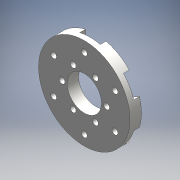
# Autodesk Inventor part: terminal-cap
Saved by Autodesk Inventor 2018 (Build 220112000, 112)
## iProperties
Created: 2026-06-13
Part Number: terminal-cap
Material: Generic
Document SubType Name: Modeling
Designer: neo
Density: 1 g/cm^3
Appearance: Default
Author: neo
Autodesk Inventor part; units mm, degrees
ref_plane "YZ Plane" through (0, 0, 0) normal (1, 0, 0) x (0, 1, 0)
ref_plane "XZ Plane" through (0, 0, 0) normal (0, 1, 0) x (-1, 0, 0)
ref_plane "XY Plane" through (0, 0, 0) normal (0, 0, 1) x (1, 0, 0)
sketch "Sketch1" plane through (0, 0, 0) normal (0, 1, 0) x (-1, 0, 0)
  circle A0 centre (0, 0) radius 30
  circle A1 centre (0, 0) radius 39 construction
  circle A2 centre (0, 0) radius 80
  circle A3 centre (39, 0) radius 5.1
  circle A4 centre (19.5, 33.775) radius 5.1
  circle A5 centre (-19.5, 33.775) radius 5.1
  circle A6 centre (-39, 0) radius 5.1
  circle A7 centre (-19.5, -33.775) radius 5.1
  circle A8 centre (19.5, -33.775) radius 5.1
  dimension "d0" = 78
  dimension "d1" = 160
  dimension "d2" = 60
  dimension "d3" = 10.2
  dimension "d6" = 360
  constraints: 8 centre point, 3 coincident, 1 horizontal alignment, 15 other
  measures "d1" diameter of A2
  measures "d2" diameter of A0
  measures "d3" diameter of A3
extrude "Extrusion1" add sketch "Sketch1" along normal blind 20
sketch "Sketch2" plane through (0, 20, 0) normal (0, 1, 0) x (1, 0, 0)
  circle A0 centre (0, 0) radius 30 construction
  circle A1 centre (-19.5, 33.775) radius 5.1 construction
  circle A2 centre (19.5, 33.775) radius 5.1 construction
  circle A3 centre (39, 0) radius 5.1 construction
  circle A4 centre (19.5, -33.775) radius 5.1 construction
  circle A5 centre (-19.5, -33.775) radius 5.1 construction
  circle A6 centre (-39, 0) radius 5.1 construction
  circle A7 centre (0, 0) radius 80 construction
  line L0 (0, -80) -> (0, 80) construction
  line L1 (-18, 80) -> (18, 80)
  line L2 (18, 80) -> (18, 44)
  line L3 (18, 44) -> (-18, 44)
  line L4 (-18, 44) -> (-18, 80)
  circle A8 centre (0, 0) radius 80 construction
  circle A9 centre (0, 62) radius 5.05
  dimension "d10" = 36
  dimension "d11" = 10.1
  dimension "d12" = 18
  dimension "d13" = 36
  constraints: 10 end point, 2 parallel, 2 point on circle, 1 centre point, 1 horizontal, 1 perpendicular, 1 point on line, 1 tangent, 1 vertical, 1 other
  measures "d10" distance between parallel lines of L2 L4
  measures "d11" diameter of A9
  measures "d12" distance from line of L1 A9.centre
  measures "d13" distance of L3.end L1.start
extrude "Extrusion2" cut sketch "Sketch2" against normal blind 10
extrude "Extrusion3" cut sketch "Sketch2" against normal through all contours A9
pattern_circular "Circular Pattern1" count 6 over 360 about axis through (0, 0, 0) along (0, 1, 0) of "Extrusion2", "Extrusion3"
body "Solid1"
